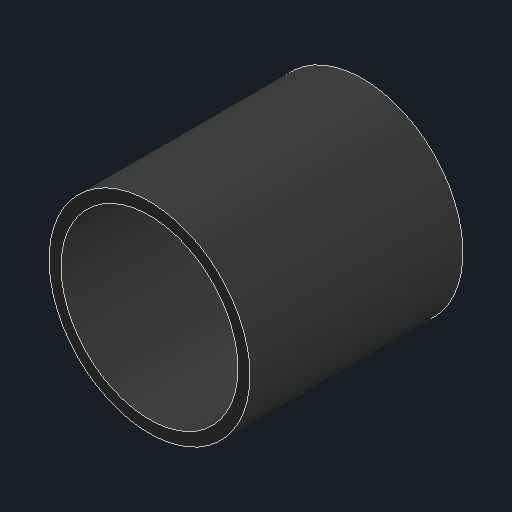
# Autodesk Inventor part: oponka
Saved by Autodesk Inventor 2023 (Build 270158000, 158)
## iProperties
Created: 2024-06-08
Part Number: oponka
Material: Rubber
Document SubType Name: Modeling
Designer: szymo
Density: 0.93 g/cm^3
Appearance: Rubber - Black
Mass: 21.8337 g
Surface Area: 165.373 cm^2
Volume: 23.4771 cm^3
Author: szymo
Autodesk Inventor part; units mm, degrees
ref_plane "YZ Plane" through (0, 0, 0) normal (1, 0, 0) x (0, 1, 0)
ref_plane "XZ Plane" through (0, 0, 0) normal (0, 1, 0) x (-1, 0, 0)
sketch "Sketch1" plane through (0, 0, 0) normal (0, 0, 1) x (1, 0, 0)
  circle A0 centre (0, 0) radius 22 projected
  circle A1 centre (0, 0) radius 25
  dimension "d0" = 50
  constraints: 1 centre point, 1 coincident
  measures "d0" diameter of A1
ref_plane "Work Plane1" through (-22, -22, -53) normal (0, 0, -1) x (0, 1, 0)
extrude "Extrusion1" add sketch "Sketch1" against normal up to surface (53 mm away)
body "Solid1"
